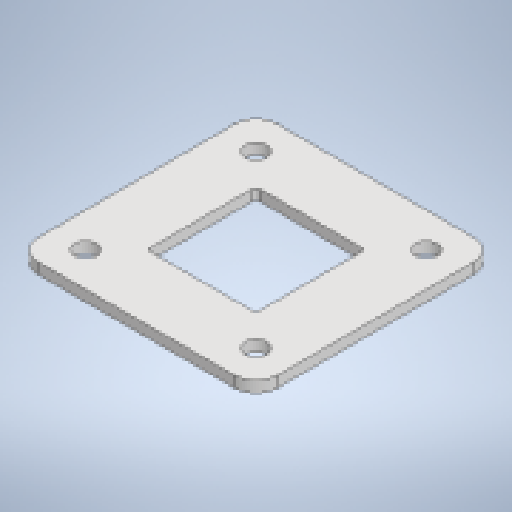
# Autodesk Inventor part: ANP 1425 FDS Way FLANGE
Saved by Autodesk Inventor 2025 (Build 290162010, 162A)
## iProperties
Created: 2025-06-24
Part Number: ANP 1425 FDS Way FLANGE
Material: Stainless Steel
Document SubType Name: Sheet Metal
Designer: user
Mass: 103.446 g
Surface Area: 101.897 cm^2
Volume: 12.9307 cm^3
Density: 8 g/cm^3
Sheet Metal Rule: AISI304 2mm Die16
Sheet Metal Width: 66,200 mm
Sheet Metal Length: 66,200 mm
Sheet Metal Area: 4382,440 mm^2
Appearance: Default
Flat Pattern Width: 6.62 cm
Flat Pattern Length: 6.62 cm
Flat Pattern Area: 43.8244 cm^2
Author: user
Autodesk Inventor part; units mm, degrees
ref_plane "YZ Plane" through (0, 0, 0) normal (1, 0, 0) x (0, 1, 0)
ref_plane "XZ Plane" through (0, 0, 0) normal (0, 1, 0) x (-1, 0, 0)
ref_plane "XY Plane" through (0, 0, 0) normal (0, 0, 1) x (1, 0, 0)
sketch "Sketch1" plane through (0, 0, 0) normal (0, 0, 1) x (1, 0, 0)
  line L0 (-33.1, -33.1) -> (33.1, -33.1)
  line L1 (33.1, -33.1) -> (33.1, 33.1)
  line L2 (33.1, 33.1) -> (-33.1, 33.1)
  line L3 (-33.1, 33.1) -> (-33.1, -33.1)
  line L4 (-33.1, -33.1) -> (33.1, 33.1) construction
  line L5 (33.1, -33.1) -> (-33.1, 33.1) construction
  line L6 (15.1, -15.1) -> (-15.1, -15.1)
  line L7 (-15.1, -15.1) -> (-15.1, 15.1)
  line L8 (-15.1, 15.1) -> (15.1, 15.1)
  line L9 (15.1, 15.1) -> (15.1, -15.1)
  line L10 (15.1, -15.1) -> (-15.1, 15.1) construction
  line L11 (-15.1, -15.1) -> (15.1, 15.1) construction
  point P0 (0, 0)
  dimension "d154" = 66.2
  dimension "d155" = 66.2
  dimension "d172" = 30.2
  dimension "d181" = 18
  measures "d154" distance of L1.end L2.end
  measures "d155" distance of L0.end L1.end
  measures "d172" distance of L7.end L8.end
  measures "d181" distance between parallel lines of L1 L9
extrude "Plate5" add sketch "Sketch1" along normal blind 3
sketch "Sketch9" plane through (0, 0, 3) normal (0, 0, 1) x (1, 0, 0)
  circle A0 centre (23.5853, -23.5853) radius 3
  line L0 (23.5853, 23.5853) -> (-23.5853, 23.5853) construction
  line L1 (-23.5853, 23.5853) -> (-23.5853, -23.5853) construction
  line L2 (-23.5853, -23.5853) -> (23.5853, -23.5853) construction
  line L3 (23.5853, -23.5853) -> (23.5853, 23.5853) construction
  line L4 (23.5853, 23.5853) -> (-23.5853, -23.5853) construction
  line L5 (-23.5853, 23.5853) -> (23.5853, -23.5853) construction
  circle A1 centre (-23.5853, -23.5853) radius 3
  circle A2 centre (23.5853, 23.5853) radius 3
  circle A3 centre (-23.5853, 23.5853) radius 3
  circle A4 centre (0, 0) radius 33.3546 construction
  line L6 (-15.1, -15.1) -> (-15.1, 15.1) projected
  line L7 (-15.1, 15.1) -> (15.1, 15.1) projected
  line L8 (15.1, 15.1) -> (15.1, -15.1) projected
  line L9 (15.1, -15.1) -> (-15.1, -15.1) projected
  line L10 (33.1, -33.1) -> (-33.1, -33.1) projected
  line L11 (33.1, 33.1) -> (33.1, -33.1) projected
  line L12 (-33.1, 33.1) -> (33.1, 33.1) projected
  line L13 (-33.1, -33.1) -> (-33.1, 33.1) projected
  dimension "d180" = 66.7092
  dimension "d174" = 6
  dimension "d182" = 12
  constraints: 12 end point, 8 coincident, 4 centre point, 3 equal radius, 2 midpoint, 2 parallel, 2 perpendicular, 1 horizontal, 3 other
  measures "d174" diameter of A0
  measures "d182" distance of L6.end L0.end
extrude "Cut2" cut sketch "Sketch9" against normal blind 3 contours A0 | A1 | A2 | A3
fillet "Corner Round1" radius 6 4 edges at (33.1, 33.1, 1.5) (-33.1, 33.1, 1.5) (-33.1, -33.1, 1.5) (33.1, -33.1, 1.5)
fillet "Corner Round2" radius 1 4 edges at (-15.1, 15.1, 1.5) (-15.1, -15.1, 1.5) (15.1, -15.1, 1.5) (15.1, 15.1, 1.5)
body "Solid3"
